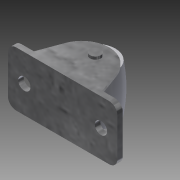
# Autodesk Inventor part: rolka_meblowa_16mm
Saved by Autodesk Inventor 2013 (Build 170138000, 138)
## iProperties
Created: 2014-04-27
Part Number: rolka_meblowa_16mm
Material: Generic
Document SubType Name: Modeling
Designer: Masta
Density: 1 g/cm^3
Author: Masta
Autodesk Inventor part; units mm, degrees
ref_plane "YZ Plane" through (0, 0, 0) normal (1, 0, 0) x (0, 1, 0)
ref_plane "XZ Plane" through (0, 0, 0) normal (0, 1, 0) x (-1, 0, 0)
ref_plane "XY Plane" through (0, 0, 0) normal (0, 0, 1) x (1, 0, 0)
sketch "Sketch1" plane through (0, 0, 0) normal (0, 0, 1) x (1, 0, 0)
  line L0 (-20, 0) -> (20, 0)
  line L1 (20, 0) -> (20, 2)
  line L2 (20, 2) -> (-20, 2)
  line L3 (-20, 2) -> (-20, 0)
  line L4 (-12.5, 2) -> (-9.3831, 10.4578)
  line L5 (9.3831, 10.4578) -> (12.5, 2)
  line L6 (0, 12) -> (0, 2) construction
  circle A0 centre (0, 12) radius 2
  arc A1 (9.3831, 10.4578) -> (-9.3831, 10.4578) centre (0, 7) ccw
  point P0 (0, 0)
  point P1 (0, 0)
  dimension "d0" = 40
  dimension "d1" = 2
  dimension "d2" = 25
  dimension "d3" = 12
  dimension "d5" = 4
  dimension "d27" = 10
  dimension "d28" = 5
  constraints: 14 end point, 2 centre point, 2 coincident, 2 midpoint, 2 parallel, 2 perpendicular, 2 point on circle, 2 point on line, 2 tangent, 1 horizontal, 1 other
  measures "d0" distance of L2.end L1.end
  measures "d1" distance of L1.end L0.end
  measures "d2" distance of L5.end L4.start
  measures "d3" distance from line of L0 L6.start
  measures "d5" diameter of A0
  measures "d27" radius of A1
  measures "d28" distance of L6.start A1.centre
extrude "Extrusion1" add sketch "Sketch1" along normal mid plane 20
extrude "Extrusion3" add sketch "Sketch1" along normal mid plane 22 contours A0
extrude "Extrusion2" cut sketch "Sketch1" along normal mid plane 18 contours L4 A1 L5 L2
sketch "Sketch2" plane through (0, 0, 0) normal (1, 0, 0) x (0, 1, 0)
  line L0 (14, -11) -> (10, -11) projected
  line L1 (10, -10) -> (0, -10) projected
  line L2 (0, -10) -> (0, 10) projected
  line L3 (0, 10) -> (10, 10) projected
  line L4 (10, 11) -> (14, 11) projected
  line L5 (12, 11) -> (12, -11)
  line L6 (14, 8.5) -> (14, -8.5)
  line L7 (14, -8.5) -> (19.2722, -8.5)
  line L8 (14, 8.5) -> (19.2722, 8.5)
  arc A0 (19.2722, -8.5) -> (19.2722, 8.5) centre (-30, 0) ccw
  line L9 (12, 0) -> (2, 0) construction
  line L10 (20, 8.5) -> (20, -8.5) construction
  line L11 (19.2722, 8.5) -> (20, 8.5) construction
  line L12 (20, -8.5) -> (19.2722, -8.5) construction
  line L13 (10, -9) -> (10, 9) projected
  line L14 (10, 9) -> (2, 9) projected
  line L15 (2, 9) -> (2, -9) projected
  line L16 (2, -9) -> (10, -9) projected
  line L17 (14, -10) -> (14, -11) projected
  line L18 (10, -11) -> (10, -10) projected
  line L19 (10, 10) -> (10, 11) projected
  line L20 (14, 11) -> (14, 10) projected
  line L21 (14, 10) -> (17, 10) projected
  line L22 (17, 10) -> (17, 9) projected
  line L23 (17, 9) -> (14, 9) projected
  line L24 (14, 9) -> (14, -9) projected
  line L25 (14, -9) -> (17, -9) projected
  line L26 (17, -9) -> (17, -10) projected
  line L27 (17, -10) -> (14, -10) projected
  point P0 (0, 0)
  dimension "d14" = 8
  dimension "d15" = 50
  dimension "d29" = 17
  constraints: 14 end point, 4 perpendicular, 2 midpoint, 2 parallel, 2 point on circle, 1 centre point, 1 collinear, 1 symmetric about line, 1 tangent, 1 other
  measures "d14" distance between parallel lines of L5 L10
  measures "d15" radius of A0
  measures "d29" distance between parallel lines of L8 L7
revolve "Revolution1" add sketch "Sketch2" angle 360 about axis through (0, 12, 11) along (0, 0, -1) contours L6 L8 A0 L7
fillet "Fillet1" radius 3 4 edges at (-20, 1, -10) (-20, 1, 10) (20, 1, 10) (20, 1, -10)
sketch "Sketch3" plane through (-17, 0, 10) normal (0, -1, 0) x (1, 0, 0)
  line L0 (37, -17) -> (37, -3) projected
  line L1 (0, 0) -> (34, 0) projected
  line L2 (-3, -3) -> (-3, -17) projected
  line L3 (34, -20) -> (0, -20) projected
  line L4 (-3, -10) -> (37, -10) construction
  line L5 (17, 0) -> (17, -20) construction
  point P0 (17, -10)
  point P1 (3, -10)
  point P2 (31, -10)
  dimension "d18" = 28
  constraints: 4 end point, 4 midpoint, 2 point on line, 1 symmetric about line
  measures "d18" distance of point (31, -10) point (3, -10)
hole "Hole1" at (-14, 0, 0) at (14, 0, 0) direction (0, 1, 0) diameter 4.5 end through all
body "Solid1"
